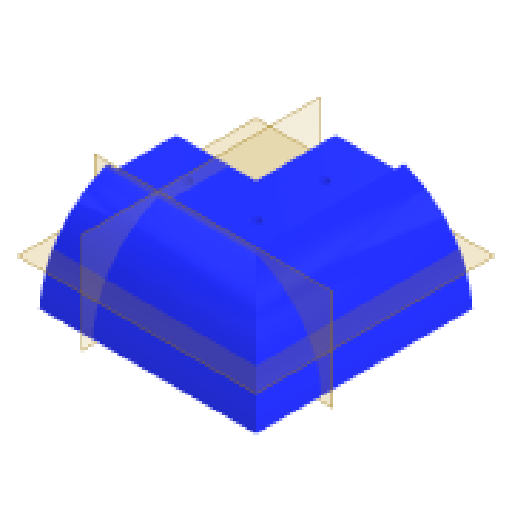
# Autodesk Inventor part: кубик
Saved by Autodesk Inventor 2023.2 (Build 272271030, 271C)
## iProperties
Created: 2025-04-24
Part Number: кубик
Material: Типовые
Document SubType Name: Modeling
Designer: Коноваленко
Density: 1 g/cm^3
Appearance: Синий — малярная краска — глянцевая
Author: Коноваленко
Autodesk Inventor part; units mm, degrees
sketch "Эскиз1" plane through (0, 0, 0) normal (0, 1, 0) x (-1, 0, 0)
  line L0 (23.2906, 28.7113) -> (-71.7094, 28.7113)
  line L1 (-71.7094, 28.7113) -> (-71.7094, -18.0259)
  line L2 (-11.7094, -31.2887) -> (23.2906, -31.2887)
  line L3 (23.2906, -31.2887) -> (23.2906, 28.7113)
  line L4 (-11.7094, -66.2887) -> (-71.7094, -66.2887)
  line L5 (-71.7094, -66.2887) -> (-71.7094, 28.7113)
  line L6 (-71.7094, 28.7113) -> (-27.2151, 28.7113)
  line L7 (-11.7094, -31.2887) -> (-11.7094, -66.2887)
  point P0 (-41.7094, -66.2887)
  dimension "d21" = 95
  dimension "d22" = 95
  dimension "d23" = 60
  dimension "d24" = 60
  constraints: 16 end point, 4 parallel, 2 horizontal, 2 perpendicular, 1 midpoint
  measures "d21" distance between parallel lines of L1 L3
  measures "d22" distance from line of point (-41.709, -66.289) L0
  measures "d23" distance between parallel lines of L5 L7
  measures "d24" distance between parallel lines of L2 L0
extrude "Выдавливание9" add sketch "Эскиз1" along normal mid plane 40
sketch "Эскиз11" plane through (-23.2906, -20, 28.7113) normal (-1, 0, 0) x (0, 0, 1)
  line L0 (0, 0) -> (0, 40) projected
  line L1 (-60, 40) -> (0, 40) projected
  line L2 (-60, 0) -> (-60, 40) projected
  line L3 (0, 0) -> (-60, 0) projected
  line L4 (-30, 40) -> (-30, 0)
  line L5 (0, 0) -> (-60, 0) projected
  arc A0 (0, 0) -> (-30, 40) centre (-44.9333, -2.4499) ccw
  point P0 (-28.7113, 20)
  constraints: 2 end point, 2 point on circle, 1 centre point, 1 midpoint, 4 other
extrude "Выдавливание11" cut sketch "Эскиз11" against normal up to surface (95 mm away) contours A0 L1 L0
sketch "Эскиз12" plane through (71.7094, 20, -66.2887) normal (0, 0, -1) x (-1, 0, 0)
  arc A0 (30, 0) -> (0, -40) centre (44.9333, -42.4499) ccw
  line L0 (0, 0) -> (60, 0) projected
  line L1 (0, -40) -> (0, 0) projected
  point P0 (71.7094, -20)
  constraints: 2 point on circle, 1 centre point, 4 other
extrude "Выдавливание12" cut sketch "Эскиз12" against normal through all
sketch "Эскиз13" plane through (0, 20, 0) normal (0, 1, 0) x (1, 0, 0)
  line L0 (41.7094, 1.2887) -> (41.7094, 66.2887) projected
  line L1 (41.7094, 66.2887) -> (11.7094, 66.2887) projected
  line L2 (11.7094, 66.2887) -> (11.7094, 31.2887) projected
  line L3 (11.7094, 31.2887) -> (-23.2906, 31.2887) projected
  line L4 (-23.2906, 31.2887) -> (-23.2906, 1.2887) projected
  line L5 (-23.2906, 1.2887) -> (41.7094, 1.2887) projected
  point P0 (0, 0)
extrude "Выдавливание13" cut sketch "Эскиз13" against normal blind 4
sketch "Эскиз14" plane through (0, 16, 0) normal (0, 1, 0) x (1, 0, 0)
  line L0 (11.7094, 66.2887) -> (41.7094, 66.2887) projected
  line L1 (26.7094, 66.2887) -> (26.7094, 16.2887) construction
  line L2 (26.7094, 16.2887) -> (-23.2906, 16.2887) construction
  line L3 (-23.2906, 1.2887) -> (-23.2906, 31.2887) projected
  line L4 (-23.2906, 31.2887) -> (11.7094, 31.2887) projected
  circle A0 centre (26.7094, 16.2887) radius 2
  circle A1 centre (26.7094, 46.2887) radius 2
  circle A2 centre (-3.2906, 16.2887) radius 2
  point P0 (0, 0)
  dimension "d35" = 15
  dimension "d37" = 20
  dimension "d39" = 20
  constraints: 4 end point, 3 centre point, 2 equal radius, 2 midpoint, 2 point on line, 1 perpendicular, 1 vertical
  measures "d35" distance between parallel lines of L2 L4
  measures "d37" distance from line of L3 A2.centre
  measures "d39" distance from line of L0 A1.centre
extrude "Выдавливание14" cut sketch "Эскиз14" against normal up to surface (36 mm away)
sketch "Эскиз15" plane through (0, -20, 0) normal (0, -1, 0) x (1, 0, 0)
  line L0 (41.7094, -66.2887) -> (46.7094, -56.2887) projected
  line L1 (26.7094, -56.2887) -> (31.7094, -66.2887) projected
  line L2 (46.7094, -56.2887) -> (26.7094, -56.2887) projected
  line L3 (11.7094, -66.2887) -> (71.7094, -66.2887) projected
  point P0 (0, 0)
extrude "Выдавливание15" cut sketch "Эскиз15" against normal blind 20
ref_plane "РабПлоскость1" through (-23.2906, -20, -66.2887) normal (-0.7071068, 0, 0.7071068) x (0, 1, 0)
mirror "Зеркальное отражение1" about plane through (-23.2906, -20, -66.2887) normal (-0.7071068, 0, 0.7071068) of "Выдавливание15"
